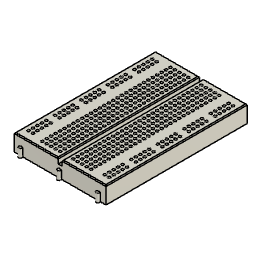
small_breadboard v1 (Autodesk Fusion 360 design; units mm, degrees)
Autodesk Fusion 360 part; units mm, degrees
(part 1 of 2)
sketch "Sketch1" plane through (0, 0, 0) normal (0, 0, 1) x (1, 0, 0)
  line L0 (26.4, -40.65) -> (-26.4, -40.65)
  line L1 (-26.4, -40.65) -> (-26.4, 40.65)
  line L2 (-26.4, 40.65) -> (26.4, 40.65)
  line L3 (26.4, 40.65) -> (26.4, -40.65)
  dimension "d1" = 52.8
  dimension "d2" = 81.3
  dimension "d3" = 40.65
  dimension "d5" = 26.4
  constraint horizontal L0
  constraint vertical L1
  constraint horizontal L2
  constraint vertical L3
  measures "d1" distance of L0.start L0.end
  measures "d2" distance of L0.start L2.end
  measures "d3" distance of origin L2
  measures "d5" distance of origin L1
extrude "Extrude1" add sketch "Sketch1" along normal blind 9.7 makes body 1
sketch "Sketch2" plane through (0, 0, 9.7) normal (0, 0, 1) x (-1, 0, 0)
  line L0 (-26.4, -40.65) -> (26.4, -40.65)
  line L1 (26.4, -40.65) -> (26.4, 40.65)
  line L2 (26.4, 40.65) -> (-26.4, 40.65)
  line L3 (-26.4, 40.65) -> (-26.4, -40.65)
  line L4 (1.1, -40.65) -> (-1.1, -40.65)
  line L5 (-1.1, -40.65) -> (-1.1, 40.65)
  line L6 (-1.1, 40.65) -> (1.1, 40.65)
  line L7 (1.1, 40.65) -> (1.1, -40.65)
  dimension "d8" = 2.2
  dimension "d9" = 81.3
  dimension "d10" = 1.1
  dimension "d11" = 2.2
  constraint horizontal L4
  constraint vertical L5
  constraint horizontal L6
  constraint vertical L7
  constraint coincident L0 L4.start
  measures "d8" distance of L4.start L4.end
  measures "d9" distance of L4.start L6.end
  measures "d10" distance of origin L5
  measures "d11" distance of L5.end L6.end
extrude "Extrude2" cut sketch "Sketch2" against normal blind 3 contours L0 L2 L4 L5 L6 L7 bodies 1
sketch "Sketch3" plane through (0, 0, 0) normal (0, 0, 1) x (1, 0, 0)
  line L0 (26.4, 40.65) -> (1.1, 40.65) construction
  line L1 (-1.1, 40.65) -> (1.1, 40.65) construction
  line L2 (-1.1, 40.65) -> (-26.4, 40.65) construction
  line L3 (-26.4, 40.65) -> (-26.4, -40.65) construction
  line L4 (26.4, -40.65) -> (26.4, 40.65) construction
  line L5 (1.1, -40.65) -> (26.4, -40.65) construction
  line L6 (1.1, -40.65) -> (-1.1, -40.65) construction
  line L7 (-26.4, -40.65) -> (-1.1, -40.65) construction
sketch "Sketch4" plane through (0, 0, 0) normal (0, 0, 1) x (1, 0, 0)
  circle A0 centre (-27, -27.3) radius 1
  line L0 (-26.4, -40.65) -> (-26.4, 40.65)
  line L1 (26.4, -40.65) -> (-26.4, -40.65)
  circle A1 centre (-27, 27.3) radius 1
  line L2 (-26.4, 40.65) -> (26.4, 40.65)
  circle A2 centre (0, -41.25) radius 1
  circle A3 centre (-22.3, -41.25) radius 1
  circle A4 centre (22.3, -41.25) radius 1
  dimension "d14" = 2
  dimension "d15" = 0.6
  dimension "d16" = 13.35
  dimension "d17" = 2
  dimension "d18" = 0.6
  dimension "d20" = 54.6
  dimension "d21" = 2
  dimension "d22" = 0.6
  dimension "d23" = 2
  dimension "d24" = 0.6
  dimension "d25" = 22.3
  dimension "d26" = 2
  dimension "d27" = 0.6
  dimension "d28" = 22.3
  measures "d14" diameter of A0
  measures "d15" distance of A0.centre L0
  measures "d16" distance of A0.centre L1
  measures "d17" diameter of A1
  measures "d18" distance of L0 A1.centre
  measures "d20" distance of A0.centre A1.centre
  measures "d21" diameter of A2
  measures "d22" distance of L1 A2.centre
  measures "d23" diameter of A3
  measures "d24" distance of L1 A3.centre
  measures "d25" distance of A2.centre A3.centre
  measures "d26" diameter of A4
  measures "d27" distance of L1 A4.centre
  measures "d28" distance of A2.centre A4.centre
extrude "Extrude3" add sketch "Sketch4" along normal blind 4.8 contours A0 L0 | L0 A1 | L1 A4 | L1 A2 | L1 A3 picked at (-26.812, -26.9871) picked at (-27.2026, 27.3104) picked at (22.6281, -41.4217) picked at (-0.0584, -41.1782) picked at (-22.3584, -41.1782) bodies 1
sketch "Sketch8" plane through (0, 0, 9.7) normal (0, 0, 1) x (-1, 0, 0)
  line L0 (-1.1, -40.65) -> (-1.1, 40.65)
  line L1 (-1.1, 40.65) -> (-26.4, 40.65)
  line L2 (-26.4, 40.65) -> (-26.4, -40.65)
  line L3 (-26.4, -40.65) -> (-1.1, -40.65)
  line L4 (0, 0) -> (26.4, 0) construction
  line L5 (-20, 0) -> (-2.5, 0)
  line L6 (0, -2.5) -> (0, -20)
  point P0 (3.8, -1.27)
  point P1 (6.34, -1.27)
  point P2 (8.88, -1.27)
  point P3 (11.42, -1.27)
  point P4 (13.96, -1.27)
  point P5 (3.8, -3.81)
  point P6 (6.34, -3.81)
  point P7 (8.88, -3.81)
  point P8 (11.42, -3.81)
  point P9 (13.96, -3.81)
  point P10 (3.8, -6.35)
  point P11 (6.34, -6.35)
  point P12 (8.88, -6.35)
  point P13 (11.42, -6.35)
  point P14 (13.96, -6.35)
  point P15 (3.8, -8.89)
  point P16 (6.34, -8.89)
  point P17 (8.88, -8.89)
  point P18 (11.42, -8.89)
  point P19 (13.96, -8.89)
  point P20 (3.8, -11.43)
  point P21 (6.34, -11.43)
  point P22 (8.88, -11.43)
  point P23 (11.42, -11.43)
  point P24 (13.96, -11.43)
  point P25 (3.8, -13.97)
  point P26 (6.34, -13.97)
  point P27 (8.88, -13.97)
  point P28 (11.42, -13.97)
  point P29 (13.96, -13.97)
  point P30 (3.8, -16.51)
  point P31 (6.34, -16.51)
  point P32 (8.88, -16.51)
  point P33 (11.42, -16.51)
  point P34 (13.96, -16.51)
  point P35 (3.8, -19.05)
  point P36 (6.34, -19.05)
  point P37 (8.88, -19.05)
  point P38 (11.42, -19.05)
  point P39 (13.96, -19.05)
  point P40 (3.8, -21.59)
  point P41 (6.34, -21.59)
  point P42 (8.88, -21.59)
  point P43 (11.42, -21.59)
  point P44 (13.96, -21.59)
  point P45 (3.8, -24.13)
  point P46 (6.34, -24.13)
  point P47 (8.88, -24.13)
  point P48 (11.42, -24.13)
  point P49 (13.96, -24.13)
  point P50 (3.8, -26.67)
  point P51 (6.34, -26.67)
  point P52 (8.88, -26.67)
  point P53 (11.42, -26.67)
  point P54 (13.96, -26.67)
  point P55 (3.8, -29.21)
  point P56 (6.34, -29.21)
  point P57 (8.88, -29.21)
  point P58 (11.42, -29.21)
  point P59 (13.96, -29.21)
  point P60 (3.8, -31.75)
  point P61 (6.34, -31.75)
  point P62 (8.88, -31.75)
  point P63 (11.42, -31.75)
  point P64 (13.96, -31.75)
  point P65 (3.8, -34.29)
  point P66 (6.34, -34.29)
  point P67 (8.88, -34.29)
  point P68 (11.42, -34.29)
  point P69 (13.96, -34.29)
  point P70 (3.8, -36.83)
  point P71 (6.34, -36.83)
  point P72 (8.88, -36.83)
  point P73 (11.42, -36.83)
  point P74 (13.96, -36.83)
  point P75 (20.71, 0)
  point P76 (20.71, 5.08)
  point P77 (23.25, 5.08)
  point P78 (20.71, 2.54)
  point P79 (23.25, 2.54)
  point P80 (23.25, 0)
  point P81 (20.71, -2.54)
  point P82 (23.25, -2.54)
  point P83 (20.71, -5.08)
  point P84 (23.25, -5.08)
  point P85 (23.25, -35.56)
  point P86 (20.71, -35.56)
  point P87 (20.71, -33.02)
  point P88 (23.25, -33.02)
  point P89 (23.25, -30.48)
  point P90 (20.71, -30.48)
  point P91 (20.71, -27.94)
  point P92 (23.25, -27.94)
  point P93 (23.25, -25.4)
  point P94 (20.71, -25.4)
  point P95 (23.25, -20.32)
  point P96 (20.71, -20.32)
  point P97 (20.71, -17.78)
  point P98 (23.25, -17.78)
  point P99 (23.25, -15.24)
  point P100 (20.71, -15.24)
  point P101 (20.71, -12.7)
  point P102 (23.25, -12.7)
  point P103 (23.25, -10.16)
  point P104 (20.71, -10.16)
  point P105 (23.25, 10.16)
  point P106 (20.71, 10.16)
  point P107 (20.71, 12.7)
  point P108 (23.25, 12.7)
  point P109 (23.25, 15.24)
  point P110 (20.71, 15.24)
  point P111 (20.71, 17.78)
  point P112 (23.25, 17.78)
  point P113 (23.25, 20.32)
  point P114 (20.71, 20.32)
  point P115 (23.25, 25.4)
  point P116 (20.71, 25.4)
  point P117 (20.71, 27.94)
  point P118 (23.25, 27.94)
  point P119 (23.25, 30.48)
  point P120 (20.71, 30.48)
  point P121 (20.71, 33.02)
  point P122 (23.25, 33.02)
  point P123 (23.25, 35.56)
  point P124 (20.71, 35.56)
  point P125 (13.96, 36.83)
  point P126 (11.42, 36.83)
  point P127 (8.88, 36.83)
  point P128 (6.34, 36.83)
  point P129 (3.8, 36.83)
  point P130 (3.8, 34.29)
  point P131 (6.34, 34.29)
  point P132 (8.88, 34.29)
  point P133 (11.42, 34.29)
  point P134 (13.96, 34.29)
  point P135 (13.96, 31.75)
  point P136 (11.42, 31.75)
  point P137 (8.88, 31.75)
  point P138 (6.34, 31.75)
  point P139 (3.8, 31.75)
  point P140 (3.8, 29.21)
  point P141 (6.34, 29.21)
  point P142 (8.88, 29.21)
  point P143 (11.42, 29.21)
  point P144 (13.96, 29.21)
  point P145 (13.96, 26.67)
  point P146 (11.42, 26.67)
  point P147 (8.88, 26.67)
  point P148 (6.34, 26.67)
  point P149 (3.8, 26.67)
  point P150 (3.8, 24.13)
  point P151 (6.34, 24.13)
  point P152 (8.88, 24.13)
  point P153 (11.42, 24.13)
  point P154 (13.96, 24.13)
  point P155 (13.96, 21.59)
  point P156 (11.42, 21.59)
  point P157 (8.88, 21.59)
  point P158 (6.34, 21.59)
  point P159 (3.8, 21.59)
  point P160 (3.8, 19.05)
  point P161 (6.34, 19.05)
  point P162 (8.88, 19.05)
  point P163 (11.42, 19.05)
  point P164 (13.96, 19.05)
  point P165 (13.96, 16.51)
  point P166 (11.42, 16.51)
  point P167 (8.88, 16.51)
  point P168 (6.34, 16.51)
  point P169 (3.8, 16.51)
  point P170 (3.8, 13.97)
  point P171 (6.34, 13.97)
  point P172 (8.88, 13.97)
  point P173 (11.42, 13.97)
  point P174 (13.96, 13.97)
  point P175 (13.96, 11.43)
  point P176 (11.42, 11.43)
  point P177 (11.42, 8.89)
  point P178 (13.96, 8.89)
  point P179 (8.88, 8.89)
  point P180 (8.88, 11.43)
  point P181 (6.34, 11.43)
  point P182 (6.34, 8.89)
  point P183 (3.8, 11.43)
  point P184 (3.8, 8.89)
  point P185 (3.8, 6.35)
  point P186 (3.8, 3.81)
  point P187 (3.8, 1.27)
  point P188 (6.34, 1.27)
  point P189 (6.34, 3.81)
  point P190 (6.34, 6.35)
  point P191 (8.88, 6.35)
  point P192 (8.88, 3.81)
  point P193 (8.88, 1.27)
  point P194 (11.42, 1.27)
  point P195 (11.42, 3.81)
  point P196 (11.42, 6.35)
  point P197 (13.96, 6.35)
  point P198 (13.96, 3.81)
  point P199 (13.96, 1.27)
  point P200 (-13.96, -36.83)
  point P201 (-11.42, -36.83)
  point P202 (-8.88, -36.83)
  point P203 (-6.34, -36.83)
  point P204 (-3.8, -36.83)
  point P205 (-3.8, -34.29)
  point P206 (-6.34, -34.29)
  point P207 (-8.88, -34.29)
  point P208 (-11.42, -34.29)
  point P209 (-13.96, -34.29)
  point P210 (-13.96, -31.75)
  point P211 (-13.96, -29.21)
  point P212 (-13.96, -26.67)
  point P213 (-11.42, -26.67)
  point P214 (-11.42, -29.21)
  point P215 (-11.42, -31.75)
  point P216 (-8.88, -31.75)
  point P217 (-6.34, -31.75)
  point P218 (-3.8, -31.75)
  point P219 (-3.8, -29.21)
  point P220 (-6.34, -29.21)
  point P221 (-8.88, -29.21)
  point P222 (-8.88, -26.67)
  point P223 (-6.34, -26.67)
  point P224 (-3.8, -26.67)
  point P225 (-3.8, -24.13)
  point P226 (-3.8, -21.59)
  point P227 (-3.8, -19.05)
  point P228 (-3.8, -16.51)
  point P229 (-3.8, -13.97)
  point P230 (-3.8, -11.43)
  point P231 (-6.34, -11.43)
  point P232 (-6.34, -13.97)
  point P233 (-6.34, -16.51)
  point P234 (-6.34, -19.05)
  point P235 (-6.34, -21.59)
  point P236 (-6.34, -24.13)
  point P237 (-8.88, -24.13)
  point P238 (-8.88, -21.59)
  point P239 (-11.42, -21.59)
  point P240 (-11.42, -24.13)
  point P241 (-13.96, -24.13)
  point P242 (-13.96, -21.59)
  point P243 (-13.96, -19.05)
  point P244 (-11.42, -19.05)
  point P245 (-8.88, -19.05)
  point P246 (-8.88, -16.51)
  point P247 (-11.42, -16.51)
  point P248 (-13.96, -16.51)
  point P249 (-13.96, -13.97)
  point P250 (-11.42, -13.97)
  point P251 (-8.88, -13.97)
  point P252 (-8.88, -11.43)
  point P253 (-11.42, -11.43)
  point P254 (-13.96, -11.43)
  point P255 (-13.96, -8.89)
  point P256 (-11.42, -8.89)
  point P257 (-8.88, -8.89)
  point P258 (-6.34, -8.89)
  point P259 (-3.8, -8.89)
  point P260 (-3.8, -6.35)
  point P261 (-6.34, -6.35)
  point P262 (-8.88, -6.35)
  point P263 (-11.42, -6.35)
  point P264 (-13.96, -6.35)
  point P265 (-13.96, -3.81)
  point P266 (-13.96, -1.27)
  point P267 (-11.42, -1.27)
  point P268 (-11.42, -3.81)
  point P269 (-8.88, -3.81)
  point P270 (-6.34, -3.81)
  point P271 (-3.8, -3.81)
  point P272 (-3.8, -1.27)
  point P273 (-6.34, -1.27)
  point P274 (-8.88, -1.27)
  point P275 (-8.88, 1.27)
  point P276 (-8.88, 3.81)
  point P277 (-8.88, 6.35)
  point P278 (-8.88, 8.89)
  point P279 (-8.88, 11.43)
  point P280 (-6.34, 11.43)
  point P281 (-3.8, 11.43)
  point P282 (-11.42, 11.43)
  point P283 (-13.96, 11.43)
  point P284 (-13.96, 8.89)
  point P285 (-13.96, 6.35)
  point P286 (-11.42, 6.35)
  point P287 (-11.42, 8.89)
  point P288 (-6.34, 8.89)
  point P289 (-6.34, 6.35)
  point P290 (-3.8, 6.35)
  point P291 (-3.8, 8.89)
  point P292 (-6.34, 3.81)
  point P293 (-6.34, 1.27)
  point P294 (-3.8, 1.27)
  point P295 (-3.8, 3.81)
  point P296 (-11.42, 3.81)
  point P297 (-13.96, 3.81)
  point P298 (-13.96, 1.27)
  point P299 (-11.42, 1.27)
  point P300 (-13.96, 13.97)
  point P301 (-13.96, 16.51)
  point P302 (-11.42, 16.51)
  point P303 (-11.42, 13.97)
  point P304 (-8.88, 13.97)
  point P305 (-8.88, 16.51)
  point P306 (-6.34, 16.51)
  point P307 (-3.8, 16.51)
  point P308 (-3.8, 13.97)
  point P309 (-6.34, 13.97)
  point P310 (-6.34, 19.05)
  point P311 (-6.34, 21.59)
  point P312 (-6.34, 24.13)
  point P313 (-6.34, 26.67)
  point P314 (-6.34, 29.21)
  point P315 (-6.34, 31.75)
  point P316 (-6.34, 34.29)
  point P317 (-6.34, 36.83)
  point P318 (-11.42, 36.83)
  point P319 (-11.42, 34.29)
  point P320 (-11.42, 31.75)
  point P321 (-11.42, 29.21)
  point P322 (-11.42, 26.67)
  point P323 (-11.42, 24.13)
  point P324 (-11.42, 21.59)
  point P325 (-11.42, 19.05)
  point P326 (-8.88, 19.05)
  point P327 (-8.88, 21.59)
  point P328 (-8.88, 24.13)
  point P329 (-13.96, 19.05)
  point P330 (-13.96, 21.59)
  point P331 (-13.96, 24.13)
  point P332 (-13.96, 26.67)
  point P333 (-13.96, 29.21)
  point P334 (-13.96, 31.75)
  point P335 (-13.96, 34.29)
  point P336 (-13.96, 36.83)
  point P337 (-3.8, 36.83)
  point P338 (-3.8, 34.29)
  point P339 (-3.8, 31.75)
  point P340 (-3.8, 29.21)
  point P341 (-3.8, 26.67)
  point P342 (-3.8, 21.59)
  point P343 (-3.8, 19.05)
  point P344 (-3.8, 24.13)
  point P345 (-8.88, 26.67)
  point P346 (-8.88, 29.21)
  point P347 (-8.88, 31.75)
  point P348 (-8.88, 34.29)
  point P349 (-8.88, 36.83)
  point P350 (-23.25, 35.56)
  point P351 (-20.71, 35.56)
  point P352 (-20.71, 33.02)
  point P353 (-23.25, 33.02)
  point P354 (-23.25, 30.48)
  point P355 (-20.71, 30.48)
  point P356 (-20.71, 27.94)
  point P357 (-23.25, 27.94)
  point P358 (-23.25, 25.4)
  point P359 (-20.71, 25.4)
  point P360 (-20.71, 20.32)
  point P361 (-23.25, 20.32)
  point P362 (-23.25, 17.78)
  point P363 (-20.71, 17.78)
  point P364 (-20.71, 15.24)
  point P365 (-23.25, 15.24)
  point P366 (-23.25, 12.7)
  point P367 (-20.71, 12.7)
  point P368 (-20.71, 10.16)
  point P369 (-23.25, 10.16)
  point P370 (-23.25, 5.08)
  point P371 (-20.71, 5.08)
  point P372 (-20.71, 2.54)
  point P373 (-23.25, 2.54)
  point P374 (-23.25, 0)
  point P375 (-20.71, 0)
  point P376 (-20.71, -2.54)
  point P377 (-23.25, -2.54)
  point P378 (-23.25, -5.08)
  point P379 (-20.71, -5.08)
  point P380 (-20.71, -10.16)
  point P381 (-23.25, -10.16)
  point P382 (-23.25, -12.7)
  point P383 (-20.71, -12.7)
  point P384 (-20.71, -15.24)
  point P385 (-23.25, -15.24)
  point P386 (-23.25, -17.78)
  point P387 (-20.71, -17.78)
  point P388 (-20.71, -20.32)
  point P389 (-23.25, -20.32)
  point P390 (-20.71, -25.4)
  point P391 (-23.25, -25.4)
  point P392 (-23.25, -27.94)
  point P393 (-20.71, -27.94)
  point P394 (-20.71, -30.48)
  point P395 (-23.25, -30.48)
  point P396 (-23.25, -33.02)
  point P397 (-20.71, -33.02)
  point P398 (-20.71, -35.56)
  point P399 (-23.25, -35.56)
  dimension "d39" = 3.8
  dimension "d40" = 1.27
  dimension "d43" = 10.16
  dimension "d44" = -35.56
  dimension "d46" = 6.75
  dimension "d49" = 2.54
  dimension "d50" = -5.08
  dimension "d53" = 0
  dimension "d54" = 30.48
  constraint coincident L4.start origin
  constraint horizontal L4
  constraint coincident L4 P75
  constraint symmetric P0 L5 P187
  constraint symmetric P1 L5 P188
  constraint symmetric P2 L5 P193
  constraint symmetric P3 L5 P194
  constraint symmetric P4 L5 P199
  constraint symmetric P5 L5 P186
  constraint symmetric P6 L5 P189
  constraint symmetric P7 L5 P192
  constraint symmetric P8 L5 P195
  constraint symmetric P9 L5 P198
  constraint symmetric P10 L5 P185
  constraint symmetric P11 L5 P190
  constraint symmetric P12 L5 P191
  constraint symmetric P13 L5 P196
  constraint symmetric P14 L5 P197
  constraint symmetric P15 L5 P184
  constraint symmetric P16 L5 P182
  constraint symmetric P17 L5 P179
  constraint symmetric P18 L5 P177
  constraint symmetric P19 L5 P178
  constraint symmetric P20 L5 P183
  constraint symmetric P21 L5 P181
  constraint symmetric P22 L5 P180
  constraint symmetric P23 L5 P176
  constraint symmetric P24 L5 P175
  constraint symmetric P25 L5 P170
  constraint symmetric P26 L5 P171
  constraint symmetric P27 L5 P172
  constraint symmetric P28 L5 P173
  constraint symmetric P29 L5 P174
  constraint symmetric P30 L5 P169
  constraint symmetric P31 L5 P168
  constraint symmetric P32 L5 P167
  constraint symmetric P33 L5 P166
  constraint symmetric P34 L5 P165
  constraint symmetric P35 L5 P160
  constraint symmetric P36 L5 P161
  constraint symmetric P37 L5 P162
  constraint symmetric P38 L5 P163
  constraint symmetric P39 L5 P164
  constraint symmetric P40 L5 P159
  constraint symmetric P41 L5 P158
  constraint symmetric P42 L5 P157
  constraint symmetric P43 L5 P156
  constraint symmetric P44 L5 P155
  constraint symmetric P45 L5 P150
  constraint symmetric P46 L5 P151
  constraint symmetric P47 L5 P152
  constraint symmetric P48 L5 P153
  constraint symmetric P49 L5 P154
  constraint symmetric P50 L5 P149
  constraint symmetric P51 L5 P148
  constraint symmetric P52 L5 P147
  constraint symmetric P53 L5 P146
  constraint symmetric P54 L5 P145
  constraint symmetric P55 L5 P140
  constraint symmetric P56 L5 P141
  constraint symmetric P57 L5 P142
  constraint symmetric P58 L5 P143
  constraint symmetric P59 L5 P144
  constraint symmetric P60 L5 P139
  constraint symmetric P61 L5 P138
  constraint symmetric P62 L5 P137
  constraint symmetric P63 L5 P136
  constraint symmetric P64 L5 P135
  constraint symmetric P65 L5 P130
  constraint symmetric P66 L5 P131
  constraint symmetric P67 L5 P132
  constraint symmetric P68 L5 P133
  constraint symmetric P69 L5 P134
  constraint symmetric P70 L5 P129
  constraint symmetric P71 L5 P128
  constraint symmetric P72 L5 P127
  constraint symmetric P73 L5 P126
  constraint symmetric P74 L5 P125
  constraint symmetric P0 L6 P272
  constraint symmetric P1 L6 P273
  constraint symmetric P2 L6 P274
  constraint symmetric P3 L6 P267
  constraint symmetric P4 L6 P266
  constraint symmetric P5 L6 P271
  constraint symmetric P6 L6 P270
  constraint symmetric P7 L6 P269
  constraint symmetric P8 L6 P268
  constraint symmetric P9 L6 P265
  constraint symmetric P10 L6 P260
  constraint symmetric P11 L6 P261
  constraint symmetric P12 L6 P262
  constraint symmetric P13 L6 P263
  constraint symmetric P14 L6 P264
  constraint symmetric P15 L6 P259
  constraint symmetric P16 L6 P258
  constraint symmetric P17 L6 P257
  constraint symmetric P18 L6 P256
  constraint symmetric P19 L6 P255
  constraint symmetric P20 L6 P230
  constraint symmetric P21 L6 P231
  constraint symmetric P22 L6 P252
  constraint symmetric P23 L6 P253
  constraint symmetric P24 L6 P254
  constraint symmetric P25 L6 P229
  constraint symmetric P26 L6 P232
  constraint symmetric P27 L6 P251
  constraint symmetric P28 L6 P250
  constraint symmetric P29 L6 P249
  constraint symmetric P30 L6 P228
  constraint symmetric P31 L6 P233
  constraint symmetric P32 L6 P246
  constraint symmetric P33 L6 P247
  constraint symmetric P34 L6 P248
  constraint symmetric P35 L6 P227
  constraint symmetric P36 L6 P234
  constraint symmetric P37 L6 P245
  constraint symmetric P38 L6 P244
  constraint symmetric P39 L6 P243
  constraint symmetric P40 L6 P226
  constraint symmetric P41 L6 P235
  constraint symmetric P42 L6 P238
  constraint symmetric P43 L6 P239
  constraint symmetric P44 L6 P242
  constraint symmetric P45 L6 P225
  constraint symmetric P46 L6 P236
  constraint symmetric P47 L6 P237
  constraint symmetric P48 L6 P240
  constraint symmetric P49 L6 P241
  constraint symmetric P50 L6 P224
  constraint symmetric P51 L6 P223
  constraint symmetric P52 L6 P222
  constraint symmetric P53 L6 P213
  constraint symmetric P54 L6 P212
  constraint symmetric P55 L6 P219
  constraint symmetric P56 L6 P220
  constraint symmetric P57 L6 P221
  constraint symmetric P58 L6 P214
  constraint symmetric P59 L6 P211
  constraint symmetric P60 L6 P218
  constraint symmetric P61 L6 P217
  constraint symmetric P62 L6 P216
  constraint symmetric P63 L6 P215
  constraint symmetric P64 L6 P210
  constraint symmetric P65 L6 P205
  constraint symmetric P66 L6 P206
  constraint symmetric P67 L6 P207
  constraint symmetric P68 L6 P208
  constraint symmetric P69 L6 P209
  constraint symmetric P70 L6 P204
  constraint symmetric P71 L6 P203
  constraint symmetric P72 L6 P202
  constraint symmetric P73 L6 P201
  constraint symmetric P74 L6 P200
  constraint symmetric P75 L6 P375
  constraint symmetric P76 L6 P371
  constraint symmetric P77 L6 P370
  constraint symmetric P78 L6 P372
  constraint symmetric P79 L6 P373
  constraint symmetric P80 L6 P374
  constraint symmetric P81 L6 P376
  constraint symmetric P82 L6 P377
  constraint symmetric P83 L6 P379
  constraint symmetric P84 L6 P378
  constraint symmetric P85 L6 P399
  constraint symmetric P86 L6 P398
  constraint symmetric P87 L6 P397
  constraint symmetric P88 L6 P396
  constraint symmetric P89 L6 P395
  constraint symmetric P90 L6 P394
  constraint symmetric P91 L6 P393
  constraint symmetric P92 L6 P392
  constraint symmetric P93 L6 P391
  constraint symmetric P94 L6 P390
  constraint symmetric P95 L6 P389
  constraint symmetric P96 L6 P388
  constraint symmetric P97 L6 P387
  constraint symmetric P98 L6 P386
  constraint symmetric P99 L6 P385
  constraint symmetric P100 L6 P384
  constraint symmetric P101 L6 P383
  constraint symmetric P102 L6 P382
  constraint symmetric P103 L6 P381
  constraint symmetric P104 L6 P380
  constraint symmetric P105 L6 P369
  constraint symmetric P106 L6 P368
  constraint symmetric P107 L6 P367
  constraint symmetric P108 L6 P366
  constraint symmetric P109 L6 P365
  constraint symmetric P110 L6 P364
  constraint symmetric P111 L6 P363
  constraint symmetric P112 L6 P362
  constraint symmetric P113 L6 P361
  constraint symmetric P114 L6 P360
  constraint symmetric P115 L6 P358
  constraint symmetric P116 L6 P359
  constraint symmetric P117 L6 P356
  constraint symmetric P118 L6 P357
  constraint symmetric P119 L6 P354
  constraint symmetric P120 L6 P355
  constraint symmetric P121 L6 P352
  constraint symmetric P122 L6 P353
  constraint symmetric P123 L6 P350
  constraint symmetric P124 L6 P351
  constraint symmetric P125 L6 P336
  constraint symmetric P126 L6 P318
  constraint symmetric P127 L6 P349
  constraint symmetric P128 L6 P317
  constraint symmetric P129 L6 P337
  constraint symmetric P130 L6 P338
  constraint symmetric P131 L6 P316
  constraint symmetric P132 L6 P348
  constraint symmetric P133 L6 P319
  constraint symmetric P134 L6 P335
  constraint symmetric P135 L6 P334
  constraint symmetric P136 L6 P320
  constraint symmetric P137 L6 P347
  constraint symmetric P138 L6 P315
  constraint symmetric P139 L6 P339
  constraint symmetric P140 L6 P340
  constraint symmetric P141 L6 P314
  constraint symmetric P142 L6 P346
  constraint symmetric P143 L6 P321
  constraint symmetric P144 L6 P333
  constraint symmetric P145 L6 P332
  constraint symmetric P146 L6 P322
  constraint symmetric P147 L6 P345
  constraint symmetric P148 L6 P313
  constraint symmetric P149 L6 P341
  constraint symmetric P150 L6 P344
  constraint symmetric P151 L6 P312
  constraint symmetric P152 L6 P328
  constraint symmetric P153 L6 P323
  constraint symmetric P154 L6 P331
  constraint symmetric P155 L6 P330
  constraint symmetric P156 L6 P324
  constraint symmetric P157 L6 P327
  constraint symmetric P158 L6 P311
  constraint symmetric P159 L6 P342
  constraint symmetric P160 L6 P343
  constraint symmetric P161 L6 P310
  constraint symmetric P162 L6 P326
  constraint symmetric P163 L6 P325
  constraint symmetric P164 L6 P329
  constraint symmetric P165 L6 P301
  constraint symmetric P166 L6 P302
  constraint symmetric P167 L6 P305
  constraint symmetric P168 L6 P306
  constraint symmetric P169 L6 P307
  constraint symmetric P170 L6 P308
  constraint symmetric P171 L6 P309
  constraint symmetric P172 L6 P304
  constraint symmetric P173 L6 P303
  constraint symmetric P174 L6 P300
  constraint symmetric P175 L6 P283
  constraint symmetric P176 L6 P282
  constraint symmetric P177 L6 P287
  constraint symmetric P178 L6 P284
  constraint symmetric P179 L6 P278
  constraint symmetric P180 L6 P279
  constraint symmetric P181 L6 P280
  constraint symmetric P182 L6 P288
  constraint symmetric P183 L6 P281
  constraint symmetric P184 L6 P291
  constraint symmetric P185 L6 P290
  constraint symmetric P186 L6 P295
  constraint symmetric P187 L6 P294
  constraint symmetric P188 L6 P293
  constraint symmetric P189 L6 P292
  constraint symmetric P190 L6 P289
  constraint symmetric P191 L6 P277
  constraint symmetric P192 L6 P276
  constraint symmetric P193 L6 P275
  constraint symmetric P194 L6 P299
  constraint symmetric P195 L6 P296
  constraint symmetric P196 L6 P286
  constraint symmetric P197 L6 P285
  constraint symmetric P198 L6 P297
  constraint symmetric P199 L6 P298
  measures "d39" horizontal distance of L4.start P0
  measures "d40" vertical distance of L4.start P0
  measures "d46" horizontal distance of P4 P75
hole "Hole1" at (-23.25, 35.56, 9.7) at (-20.71, 35.56, 9.7) at (-20.71, 33.02, 9.7) at (-20.71, 30.48, 9.7) at (-20.71, 27.94, 9.7) at (-20.71, 25.4, 9.7) at (-23.25, 25.4, 9.7) at (-23.25, 27.94, 9.7) at (-23.25, 30.48, 9.7) at (-23.25, 33.02, 9.7) at (20.71, 5.08, 9.7) at (23.25, 5.08, 9.7) at (23.25, 2.54, 9.7) at (20.71, 2.54, 9.7) at (20.71, 0, 9.7) at (23.25, 0, 9.7) at (23.25, -2.54, 9.7) at (20.71, -2.54, 9.7) at (20.71, -5.08, 9.7) at (23.25, -5.08, 9.7) at (23.25, -10.16, 9.7) at (20.71, -10.16, 9.7) at (20.71, -12.7, 9.7) at (23.25, -12.7, 9.7) at (23.25, -15.24, 9.7) at (20.71, -15.24, 9.7) at (20.71, -17.78, 9.7) at (23.25, -17.78, 9.7) at (23.25, -20.32, 9.7) at (20.71, -20.32, 9.7) at (20.71, -25.4, 9.7) at (23.25, -25.4, 9.7) at (23.25, -27.94, 9.7) at (23.25, -30.48, 9.7) at (23.25, -33.02, 9.7) at (23.25, -35.56, 9.7) at (20.71, -35.56, 9.7) at (20.71, -33.02, 9.7) at (20.71, -30.48, 9.7) at (20.71, -27.94, 9.7) at (20.71, 10.16, 9.7) at (23.25, 10.16, 9.7) at (23.25, 12.7, 9.7) at (20.71, 12.7, 9.7) at (20.71, 15.24, 9.7) at (23.25, 15.24, 9.7) at (23.25, 17.78, 9.7) at (20.71, 17.78, 9.7) at (20.71, 20.32, 9.7) at (23.25, 20.32, 9.7) at (23.25, 25.4, 9.7) at (20.71, 25.4, 9.7) at (20.71, 27.94, 9.7) at (23.25, 27.94, 9.7) at (23.25, 30.48, 9.7) at (20.71, 30.48, 9.7) at (20.71, 33.02, 9.7) at (23.25, 33.02, 9.7) at (23.25, 35.56, 9.7) at (20.71, 35.56, 9.7) at (-20.71, 20.32, 9.7) at (-23.25, 20.32, 9.7) at (-23.25, 17.78, 9.7) at (-20.71, 17.78, 9.7) at (-20.71, 15.24, 9.7) at (-23.25, 15.24, 9.7) at (-23.25, 12.7, 9.7) at (-20.71, 12.7, 9.7) at (-20.71, 10.16, 9.7) at (-23.25, 10.16, 9.7) at (-20.71, 5.08, 9.7) at (-20.71, 2.54, 9.7) at (-20.71, 0, 9.7) at (-20.71, -2.54, 9.7) at (-20.71, -5.08, 9.7) at (-23.25, -5.08, 9.7) at (-23.25, -2.54, 9.7) at (-23.25, 0, 9.7) at (-23.25, 2.54, 9.7) at (-23.25, 5.08, 9.7) at (-20.71, -10.16, 9.7) at (-20.71, -12.7, 9.7) at (-20.71, -15.24, 9.7) at (-20.71, -17.78, 9.7) at (-20.71, -20.32, 9.7) at (-23.25, -20.32, 9.7) at (-23.25, -17.78, 9.7) at (-23.25, -15.24, 9.7) at (-23.25, -12.7, 9.7) at (-23.25, -10.16, 9.7) at (-23.25, -25.4, 9.7) at (-23.25, -27.94, 9.7) at (-23.25, -30.48, 9.7) at (-23.25, -33.02, 9.7) at (-23.25, -35.56, 9.7) at (-20.71, -35.56, 9.7) at (-20.71, -33.02, 9.7) at (-20.71, -30.48, 9.7) at (-20.71, -27.94, 9.7) at (-20.71, -25.4, 9.7) at (-13.96, -36.83, 9.7) at (-11.42, -36.83, 9.7) at (-8.88, -36.83, 9.7) at (-6.34, -36.83, 9.7) at (-3.8, -36.83, 9.7) at (-6.34, -34.29, 9.7) at (-8.88, -31.75, 9.7) at (-11.42, -29.21, 9.7) at (-13.96, -26.67, 9.7) at (-13.96, -29.21, 9.7) at (-13.96, -31.75, 9.7) at (-13.96, -34.29, 9.7) at (-11.42, -34.29, 9.7) at (-8.88, -34.29, 9.7) at (-11.42, -31.75, 9.7) at (-11.42, -26.67, 9.7) at (-8.88, -26.67, 9.7) at (-6.34, -26.67, 9.7) at (-3.8, -26.67, 9.7) at (-3.8, -29.21, 9.7) at (-3.8, -31.75, 9.7) at (-3.8, -34.29, 9.7) at (-6.34, -31.75, 9.7) at (-6.34, -29.21, 9.7) at (-8.88, -29.21, 9.7) at (-13.96, -24.13, 9.7) at (-11.42, -21.59, 9.7) at (-8.88, -19.05, 9.7) at (-6.34, -16.51, 9.7) at (-3.8, -13.97, 9.7) at (-3.8, -16.51, 9.7) at (-3.8, -19.05, 9.7) at (-3.8, -21.59, 9.7) at (-3.8, -24.13, 9.7) at (-6.34, -24.13, 9.7) at (-8.88, -24.13, 9.7) at (-11.42, -24.13, 9.7) at (-8.88, -21.59, 9.7) at (-6.34, -19.05, 9.7) at (-6.34, -21.59, 9.7) at (-13.96, -21.59, 9.7) at (-13.96, -19.05, 9.7) at (-11.42, -19.05, 9.7) at (-13.96, -16.51, 9.7) at (-11.42, -16.51, 9.7) at (-8.88, -16.51, 9.7) at (-6.34, -13.97, 9.7) at (-8.88, -13.97, 9.7) at (-11.42, -13.97, 9.7) at (-13.96, -13.97, 9.7) at (-13.96, -11.43, 9.7) at (-11.42, -11.43, 9.7) at (-8.88, -11.43, 9.7) at (-6.34, -11.43, 9.7) at (-3.8, -11.43, 9.7) at (-3.8, -8.89, 9.7) at (-3.8, -6.35, 9.7) at (-3.8, -1.27, 9.7) at (-3.8, -3.81, 9.7) at (-6.34, -1.27, 9.7) at (-6.34, -3.81, 9.7) at (-6.34, -6.35, 9.7) at (-6.34, -8.89, 9.7) at (-8.88, -8.89, 9.7) at (-8.88, -6.35, 9.7) at (-8.88, -3.81, 9.7) at (-8.88, -1.27, 9.7) at (-11.42, -1.27, 9.7) at (-11.42, -3.81, 9.7) at (-11.42, -8.89, 9.7) at (-11.42, -6.35, 9.7) at (-13.96, -8.89, 9.7) at (-13.96, -3.81, 9.7) at (-13.96, -6.35, 9.7) at (-13.96, -1.27, 9.7) at (-13.96, 1.27, 9.7) at (-11.42, 3.81, 9.7) at (-13.96, 3.81, 9.7) at (-11.42, 1.27, 9.7) at (-8.88, 3.81, 9.7) at (-8.88, 1.27, 9.7) at (-6.34, 1.27, 9.7) at (-6.34, 3.81, 9.7) at (-3.8, 3.81, 9.7) at (-3.8, 1.27, 9.7) at (-3.8, 6.35, 9.7) at (-3.8, 8.89, 9.7) at (-3.8, 11.43, 9.7) at (-3.8, 13.97, 9.7) at (-3.8, 16.51, 9.7) at (-3.8, 19.05, 9.7) at (-3.8, 21.59, 9.7) at (-3.8, 24.13, 9.7) at (-3.8, 26.67, 9.7) at (-3.8, 29.21, 9.7) at (-3.8, 31.75, 9.7) at (-3.8, 34.29, 9.7) at (-3.8, 36.83, 9.7) at (-6.34, 36.83, 9.7) at (-6.34, 34.29, 9.7) at (-6.34, 31.75, 9.7) at (-6.34, 29.21, 9.7) at (-6.34, 26.67, 9.7) at (-6.34, 24.13, 9.7) at (-6.34, 21.59, 9.7) at (-6.34, 19.05, 9.7) at (-6.34, 16.51, 9.7) at (-6.34, 13.97, 9.7) at (-6.34, 11.43, 9.7) at (-6.34, 8.89, 9.7) at (-6.34, 6.35, 9.7) at (-8.88, 6.35, 9.7) at (-11.42, 6.35, 9.7) at (-13.96, 6.35, 9.7) at (-13.96, 8.89, 9.7) at (-11.42, 8.89, 9.7) at (-8.88, 8.89, 9.7) at (-8.88, 11.43, 9.7) at (-11.42, 11.43, 9.7) at (-13.96, 11.43, 9.7) at (-13.96, 13.97, 9.7) at (-13.96, 16.51, 9.7) at (-13.96, 19.05, 9.7) at (-13.96, 21.59, 9.7) at (-13.96, 24.13, 9.7) at (-13.96, 26.67, 9.7) at (-13.96, 29.21, 9.7) at (-13.96, 31.75, 9.7) at (-13.96, 34.29, 9.7) at (-13.96, 36.83, 9.7) at (-11.42, 36.83, 9.7) at (-8.88, 36.83, 9.7) at (-8.88, 34.29, 9.7) at (-11.42, 34.29, 9.7) at (-11.42, 31.75, 9.7) at (-8.88, 31.75, 9.7) at (-8.88, 29.21, 9.7) at (-11.42, 29.21, 9.7) at (-11.42, 26.67, 9.7) at (-11.42, 24.13, 9.7) at (-8.88, 24.13, 9.7) at (-8.88, 26.67, 9.7) at (-8.88, 21.59, 9.7) at (-11.42, 21.59, 9.7) at (-11.42, 19.05, 9.7) at (-8.88, 19.05, 9.7) at (-8.88, 16.51, 9.7) at (-11.42, 16.51, 9.7) at (-11.42, 13.97, 9.7) at (-8.88, 13.97, 9.7) at (3.8, 36.83, 9.7) at (6.34, 36.83, 9.7) at (8.88, 36.83, 9.7) at (11.42, 36.83, 9.7) at (13.96, 36.83, 9.7) at (13.96, 34.29, 9.7) at (11.42, 34.29, 9.7) at (8.88, 34.29, 9.7) at (6.34, 34.29, 9.7) at (3.8, 34.29, 9.7) at (3.8, -36.83, 9.7) at (6.34, -36.83, 9.7) at (8.88, -36.83, 9.7) at (11.42, -36.83, 9.7) at (13.96, -36.83, 9.7) at (13.96, -34.29, 9.7) at (11.42, -34.29, 9.7) at (8.88, -34.29, 9.7) at (6.34, -34.29, 9.7) at (3.8, -34.29, 9.7) at (3.8, -31.75, 9.7) at (6.34, -31.75, 9.7) at (8.88, -31.75, 9.7) at (11.42, -31.75, 9.7) at (13.96, -31.75, 9.7) at (13.96, -29.21, 9.7) at (13.96, -26.67, 9.7) at (13.96, -24.13, 9.7) at (11.42, -24.13, 9.7) at (11.42, -26.67, 9.7) at (11.42, -29.21, 9.7) at (8.88, -29.21, 9.7) at (8.88, -26.67, 9.7) at (8.88, -24.13, 9.7) at (6.34, -24.13, 9.7) at (6.34, -26.67, 9.7) at (6.34, -29.21, 9.7) at (3.8, -29.21, 9.7) at (3.8, -26.67, 9.7) at (3.8, -24.13, 9.7) at (3.8, -21.59, 9.7) at (6.34, -21.59, 9.7) at (8.88, -21.59, 9.7) at (11.42, -21.59, 9.7) at (13.96, -21.59, 9.7) at (3.8, 31.75, 9.7) at (6.34, 31.75, 9.7) at (8.88, 31.75, 9.7) at (11.42, 31.75, 9.7) at (13.96, 31.75, 9.7) at (13.96, 29.21, 9.7) at (11.42, 29.21, 9.7) at (8.88, 29.21, 9.7) at (6.34, 29.21, 9.7) at (3.8, 29.21, 9.7) at (3.8, 26.67, 9.7) at (3.8, 24.13, 9.7) at (3.8, 21.59, 9.7) at (3.8, 19.05, 9.7) at (6.34, 19.05, 9.7) at (6.34, 21.59, 9.7) at (6.34, 24.13, 9.7) at (6.34, 26.67, 9.7) at (8.88, 26.67, 9.7) at (11.42, 26.67, 9.7) at (13.96, 26.67, 9.7) at (13.96, 24.13, 9.7) at (11.42, 24.13, 9.7) at (8.88, 24.13, 9.7) at (8.88, 21.59, 9.7) at (8.88, 19.05, 9.7) at (11.42, 19.05, 9.7) at (11.42, 21.59, 9.7) at (13.96, 21.59, 9.7) at (13.96, 19.05, 9.7) at (13.96, 16.51, 9.7) at (11.42, 16.51, 9.7) at (8.88, 16.51, 9.7) at (6.34, 16.51, 9.7) at (3.8, 16.51, 9.7) at (3.8, 13.97, 9.7) at (6.34, 13.97, 9.7) at (8.88, 13.97, 9.7) at (11.42, 13.97, 9.7) at (13.96, 13.97, 9.7) at (13.96, 11.43, 9.7) at (11.42, 11.43, 9.7) at (8.88, 11.43, 9.7) at (6.34, 11.43, 9.7) at (3.8, 11.43, 9.7) at (3.8, 8.89, 9.7) at (3.8, 6.35, 9.7) at (3.8, 3.81, 9.7) at (3.8, 1.27, 9.7) at (3.8, -1.27, 9.7) at (3.8, -3.81, 9.7) at (3.8, -6.35, 9.7) at (3.8, -8.89, 9.7) at (3.8, -11.43, 9.7) at (3.8, -13.97, 9.7) at (3.8, -16.51, 9.7) at (3.8, -19.05, 9.7) at (13.96, -19.05, 9.7) at (13.96, -16.51, 9.7) at (13.96, -13.97, 9.7) at (13.96, -11.43, 9.7) at (13.96, -8.89, 9.7) at (13.96, -6.35, 9.7) at (13.96, -1.27, 9.7) at (13.96, -3.81, 9.7) at (13.96, 1.27, 9.7) at (13.96, 3.81, 9.7) at (13.96, 6.35, 9.7) at (13.96, 8.89, 9.7) at (11.42, -19.05, 9.7) at (8.88, -19.05, 9.7) at (6.34, -19.05, 9.7) at (6.34, -16.51, 9.7) at (8.88, -16.51, 9.7) at (11.42, -16.51, 9.7) at (11.42, -13.97, 9.7) at (8.88, -13.97, 9.7) at (6.34, -13.97, 9.7) at (6.34, -11.43, 9.7) at (8.88, -11.43, 9.7) at (11.42, -11.43, 9.7) at (11.42, -8.89, 9.7) at (8.88, -8.89, 9.7) at (6.34, -8.89, 9.7) at (6.34, -6.35, 9.7) at (8.88, -6.35, 9.7) at (11.42, -6.35, 9.7) at (11.42, -3.81, 9.7) at (8.88, -3.81, 9.7) at (6.34, -3.81, 9.7) at (6.34, 8.89, 9.7) at (8.88, 8.89, 9.7) at (11.42, 8.89, 9.7) at (6.34, 6.35, 9.7) at (8.88, 6.35, 9.7) at (11.42, 6.35, 9.7) at (6.34, 3.81, 9.7) at (6.34, 1.27, 9.7) at (6.34, -1.27, 9.7) at (8.88, -1.27, 9.7) at (11.42, -1.27, 9.7) at (11.42, 1.27, 9.7) at (11.42, 3.81, 9.7) at (8.88, 3.81, 9.7) at (8.88, 1.27, 9.7) direction (0, 0, -1) diameter 1.524 depth 7 tip angle 180 bodies 1
chamfer "Chamfer1" distance 0.5 angle 45 8 edges at (-26.4, 0, 9.7) (-13.75, 40.65, 9.7) (13.75, 40.65, 9.7) (-13.75, -40.65, 9.7) (1.1, 0, 9.7) (-1.1, 0, 9.7) (13.75, -40.65, 9.7) (26.4, 0, 9.7) on bodies 1
sketch "Sketch9" plane through (0, 0, 0) normal (1, 0, 0) x (0, 1, 0)
sketch "Sketch10" plane through (0, 0, 0) normal (0, 0, 1) x (1, 0, 0)
  line L0 (30.5, -45) -> (-30.5, -45)
  line L1 (-30.5, -45) -> (-30.5, 45)
  line L2 (-30.5, 45) -> (30.5, 45)
  line L3 (30.5, 45) -> (30.5, -45)
  line L4 (30.5, -45) -> (-30.5, 45) construction
  line L5 (-30.5, -45) -> (30.5, 45) construction
  dimension "d59" = 61
  dimension "d60" = 90
  constraint horizontal L0
  constraint perpendicular L0 L1
  constraint parallel L0 L2
  constraint parallel L1 L3
  constraint coincident L4 origin
  constraint coincident L5 origin
  measures "d59" distance of L1.end L2.end
  measures "d60" distance of L0.end L1.end
sketch "Sketch1 (2)" plane through (0, 0, 0) normal (0, 0, 1) x (1, 0, 0) in component "Component"
  line L0 (30.5, -45) -> (-30.5, -45)
  line L1 (-30.5, -45) -> (-30.5, 45)
  line L2 (-30.5, 45) -> (30.5, 45)
  line L3 (30.5, 45) -> (30.5, -45)
  line L4 (30.5, -45) -> (-30.5, 45) construction
  line L5 (-30.5, -45) -> (30.5, 45) construction
  dimension "d63" = 61
  dimension "d64" = 90
  constraint horizontal L0
  constraint perpendicular L0 L1
  constraint parallel L0 L2
  constraint parallel L1 L3
  constraint coincident L4 origin
  constraint coincident L5 origin
  measures "d63" distance of L1.end L2.end
  measures "d64" distance of L0.end L1.end
extrude "Extrude1'" add sketch "Sketch1 (2)" along normal blind 21 separate body makes body 2 in component "Component"
move_body "Move1" bodies 1 to x (1, 0, 0) y (0, 1, 0) z (0, 0, 1) at (0, 2.5, 0)
move_body "Move2" bodies 1 to x (1, 0, 0) y (0, 1, 0) z (0, 0, 1) at (0, 0, 2.5)
move_body "Move3" bodies 1 to x (1, 0, 0) y (0, 1, 0) z (0, 0, 1) at (0, -1, 0)
move_body "Move4" bodies 1 to x (1, 0, 0) y (0, 1, 0) z (0, 0, 1) at (0.75, 0, 0)
sketch "Sketch11" plane through (0, 0, 0) normal (0, 1, 0) x (1, 0, 0)
sketch "Sketch12" plane through (0, 45, 0) normal (0, 1, 0) x (-1, 0, 0)
  line L0 (-28, 2.5) -> (28, 2.5)
  line L1 (28, 2.5) -> (28, 19.5)
  line L2 (28, 19.5) -> (-28, 19.5)
  line L3 (-28, 19.5) -> (-28, 2.5)
  line L4 (5.4131, 19.081) -> (-5.1305, 19.081)
  line L5 (-5.1305, 19.081) -> (-5.1305, 16.0289)
  line L6 (-5.1305, 16.0289) -> (5.4131, 16.0289)
  line L7 (5.4131, 16.0289) -> (5.4131, 19.081)
  line L8 (5.4131, 19.081) -> (-5.1305, 16.0289) construction
  line L9 (-5.1305, 19.081) -> (5.4131, 16.0289) construction
  point P0 (0.1413, 17.555)
  dimension "d77" = 10.5436
  dimension "d78" = 3.0521
  constraint horizontal L4
  constraint perpendicular L4 L5
  constraint parallel L4 L6
  constraint parallel L5 L7
  constraint coincident L8 P0
  constraint coincident L9 P0
  measures "d77" distance of L5.end L6.end
  measures "d78" distance of L4.end L5.end
sketch "Sketch13" plane through (0, 0, 22) normal (0, 0, 1) x (-1, 0, 0)
  line L0 (28, 42.5) -> (-28, 42.5)
  line L1 (-28, 42.5) -> (-28, -42.5)
  line L2 (-28, -42.5) -> (28, -42.5)
  line L3 (28, -42.5) -> (28, 42.5)
  line L4 (15, 20) -> (-15, 20)
  line L5 (-15, 20) -> (-15, 35)
  line L6 (-15, 35) -> (15, 35)
  line L7 (15, 35) -> (15, 20)
  dimension "d81" = 30
  dimension "d82" = 15
  constraint horizontal L4
  constraint vertical L5
  constraint horizontal L6
  constraint vertical L7
  measures "d81" distance of L4.start L4.end
  measures "d82" distance of L4.start L6.end